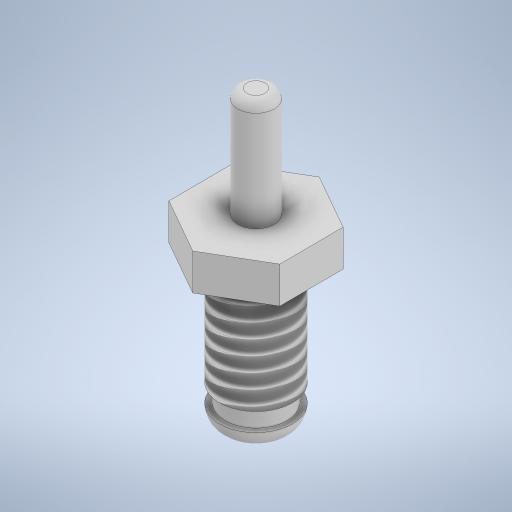
# Autodesk Inventor part: temperature sensor
Saved by Autodesk Inventor 2023 (Build 270158000, 158)
## iProperties
Created: 2022-08-26
Part Number: temperature sensor
Material: Generic
Document SubType Name: Modeling
Designer: station
Density: 1 g/cm^3
Appearance: Default
Author: station
Autodesk Inventor part; units mm, degrees
ref_plane "YZ Plane" through (0, 0, 0) normal (1, 0, 0) x (0, 1, 0)
ref_plane "XZ Plane" through (0, 0, 0) normal (0, 1, 0) x (-1, 0, 0)
ref_plane "XY Plane" through (0, 0, 0) normal (0, 0, 1) x (1, 0, 0)
sketch "Sketch1" plane through (0, 0, 0) normal (0, 0, 1) x (1, 0, 0)
  line L0 (0, 0) -> (0.5, 0)
  line L1 (1, 1) -> (1, 4)
  line L2 (1, 4) -> (0, 4)
  line L3 (0, 4) -> (0, 0)
  arc A0 (0.5, 0) -> (1, 0.5) centre (0.5, 0.5) ccw
  line L4 (1, 0.5) -> (0.85, 0.5)
  line L5 (0.85, 0.5) -> (0.85, 1)
  line L6 (0.85, 1) -> (1, 1)
  point P0 (1, 0)
  dimension "d0" = 1
  dimension "d1" = 4
  dimension "d2" = 0.5
  dimension "d6" = 0.15
  dimension "d7" = 0.5
  constraints: 14 end point, 5 perpendicular, 2 horizontal, 2 point on circle, 2 point on line, 2 tangent, 1 centre point
  measures "d0" distance of L0.start point (1, 0)
  measures "d1" distance of L1.end point (1, 0)
  measures "d2" radius of A0
  measures "d6" distance of L4.start L4.end
  measures "d7" distance of L4.end L5.end
revolve "Revolution1" add sketch "Sketch1" angle 360 about axis through (0, 4, 0) along (0, -1, 0)
thread "Thread1" size "M2x0.4" class "6g" standard "ISO Metric profile" length 3
sketch "Sketch2" plane through (0, 4, 0) normal (0, 1, 0) x (1, 0, 0)
  circle A0 centre (0, 0) radius 0.5 projected
  circle A1 centre (0, 0) radius 1.75 construction
  line L0 (-1.5102, -0.8843) -> (-1.5209, 0.8657)
  line L1 (-1.5209, 0.8657) -> (-0.0107, 1.75)
  line L2 (-0.0107, 1.75) -> (1.5102, 0.8843)
  line L3 (1.5102, 0.8843) -> (1.5209, -0.8657)
  line L4 (1.5209, -0.8657) -> (0.0107, -1.75)
  line L5 (0.0107, -1.75) -> (-1.5102, -0.8843)
  dimension "d8" = 3.5
  constraints: 12 end point, 2 coincident, 16 other
extrude "Extrusion1" add sketch "Sketch2" along normal blind 1
extrude "Extrusion2" add sketch "Sketch2" along normal blind 4 contours A0
fillet "Fillet1" radius 0.25 1 edges at (-0.5, 8, 0)
body "Solid1"
